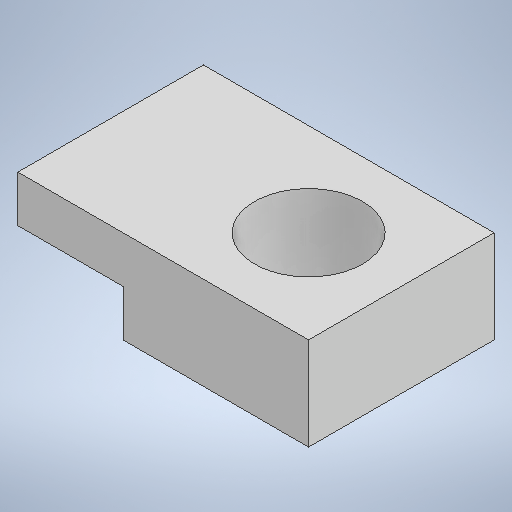
# Autodesk Inventor part: 12Vnub
Saved by Autodesk Inventor 2025 (Build 290162000, 162)
## iProperties
Created: 2025-05-31
Part Number: 12Vnub
Material: Generic
Document SubType Name: Modeling
Designer: ethan
Density: 1 g/cm^3
Appearance: Default
Author: ethan
Autodesk Inventor part; units mm, degrees
ref_plane "YZ Plane" through (0, 0, 0) normal (1, 0, 0) x (0, 1, 0)
ref_plane "XZ Plane" through (0, 0, 0) normal (0, 1, 0) x (-1, 0, 0)
ref_plane "XY Plane" through (0, 0, 0) normal (0, 0, 1) x (1, 0, 0)
sketch "Sketch1" plane through (0, 0, 0) normal (0, 1, 0) x (-1, 0, 0)
  line L0 (0, 0) -> (6, 0)
  line L1 (6, 0) -> (6, -6)
  line L2 (6, -6) -> (0, -6)
  line L3 (0, -6) -> (0, 0)
  circle A0 centre (3, -3) radius 1.75
  dimension "d0" = 6
  dimension "d1" = 6
  dimension "d2" = 3.5
  constraints: 8 end point, 2 parallel, 1 centre point, 1 horizontal, 1 perpendicular
  measures "d0" distance of L1.end L2.end
  measures "d1" distance of L0.end L1.end
  measures "d2" diameter of A0
extrude "Extrusion1" add sketch "Sketch1" along normal blind 1.5
sketch "Sketch2" plane through (0, 1.5, 0) normal (0, 1, 0) x (1, 0, 0)
  line L0 (0, 6) -> (-6, 6) projected
  line L1 (-6, 6) -> (-6, 0) projected
  line L2 (-6, 0) -> (0, 0) projected
  line L3 (0, 0) -> (0, 6) projected
  circle A0 centre (-3, 3) radius 1.75 projected
  line L4 (-6, 0) -> (-9.4, 0)
  line L5 (-9.4, 0) -> (-9.4, 6)
  line L6 (-9.4, 6) -> (-6, 6)
  line L7 (-6, 6) -> (-6, 0)
  dimension "d5" = 3.4
  constraints: 8 end point, 2 parallel, 1 horizontal, 1 perpendicular
  measures "d5" distance of L5.end L6.end
extrude "Extrusion2" add sketch "Sketch2" along normal blind 1.5
body "Solid1"
